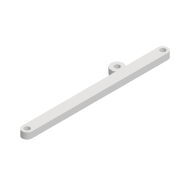
# Autodesk Inventor part: Part_2
Saved by Autodesk Inventor 2022 (Build 260153000, 153)
## iProperties
Created: 2022-04-22
Part Number: Part_2
Material: Generic
Document SubType Name: Modeling
Designer: dell
Density: 1 g/cm^3
Appearance: Default
Mass: 4.19278 g
Surface Area: 29.5472 cm^2
Volume: 4.19278 cm^3
Author: dell
Autodesk Inventor part; units mm, degrees
ref_plane "YZ Plane" through (0, 0, 0) normal (1, 0, 0) x (0, 1, 0)
ref_plane "XZ Plane" through (0, 0, 0) normal (0, 1, 0) x (-1, 0, 0)
ref_plane "XY Plane" through (0, 0, 0) normal (0, 0, 1) x (1, 0, 0)
sketch "Sketch1" plane through (0, 0, 0) normal (0, 1, 0) x (-1, 0, 0)
  line L0 (0, 0) -> (0, -110) construction
  line L1 (4, 0) -> (4, -110)
  line L2 (-4, -110) -> (-4, 0)
  arc A0 (4, 0) -> (-4, 0) centre (0, 0) ccw
  arc A1 (-4, -110) -> (4, -110) centre (0, -110) ccw
  circle A2 centre (0, 0) radius 2.1
  circle A3 centre (0, -110) radius 2.1
  circle A4 centre (7, -80) radius 2.1
  circle A5 centre (7, -80) radius 5
  point P0 (0, -55)
  point P1 (4, -76)
  point P2 (4, -84)
  dimension "d0" = 110
  dimension "d1" = 8
  dimension "d2" = 4.2
  dimension "d3" = 4.2
  dimension "d6" = 4.2
  dimension "d9" = 80
  dimension "d10" = 3
  dimension "d11" = 10
  constraints: 8 end point, 6 centre point, 4 point on circle, 4 tangent, 3 coincident, 1 midpoint, 1 parallel, 1 vertical
  measures "d0" distance of L0.end L0.start
  measures "d1" distance between parallel lines of L2 L1
  measures "d2" diameter of A2
  measures "d3" diameter of A3
  measures "d6" diameter of A4
  measures "d9" vertical distance of L0.start A4.centre
  measures "d10" distance from line of L1 A4.centre
  measures "d11" diameter of A5
extrude "Extrusion1" add sketch "Sketch1" along normal blind 5
body "Solid1"
